leg_screw (Autodesk Fusion 360 design; units mm, degrees)
Autodesk Fusion 360 part; units mm, degrees
sketch "Sketch1" plane through (0, 0, 0) normal (0, 1, 0) x (1, 0, 0)
  circle A0 centre (0, 0) radius 10
  dimension "d1" = 20
  constraint coincident A0.centre origin
  measures "d1" diameter of A0
extrude "Extrude1" add sketch "Sketch1" along normal blind 3
sketch "Sketch2" plane through (0, 0, 0) normal (0, -1, 0) x (1, 0, 0)
  circle A0 centre (0, 0) radius 10
  circle A1 centre (0, 0) radius 4
  dimension "d4" = 8
  constraint coincident A0.centre A1.centre
  measures "d4" diameter of A1
extrude "Extrude2" add sketch "Sketch2" along normal blind 20 contours A1
thread "Thread1" "ISO Metric profile 8.0 M8x1.25 6g" major diameter 7.866 minor diameter 6.4455 pitch 1.25 angle 60 modelled right hand crest width 0.1833 on face at (3.995, -13.3333, -0.1994) crest through (3.933, 0.3125, 0)
sketch "Sketch4" plane through (0, 0, 0) normal (0, 0, 1) x (1, 0, 0)
  line L0 (-10, 3) -> (10, 3)
  line L1 (5, 3) -> (-5, 3)
  line L2 (-5, 3) -> (-5, 1.6)
  line L3 (-5, 1.6) -> (5, 1.6)
  line L4 (5, 1.6) -> (5, 3)
  dimension "d9" = 5
  dimension "d10" = 5
  dimension "d11" = 1.4
  constraint horizontal L0
  constraint horizontal L1
  constraint vertical L2
  constraint horizontal L3
  constraint vertical L4
  constraint coincident L0 L1.start
  measures "d9" horizontal distance of origin L1.end
  measures "d10" horizontal distance of origin L1.start
  measures "d11" distance of L1.end L2.end
extrude "Extrude3" cut sketch "Sketch4" along normal mid plane 1.5
pattern_circular "C-Pattern1" count 3 over 180 about axis through (0, 1.75, 0) along (0, 1, 0) of "Extrude3"
equation "d10 = d9"
equation "d12 = ( 1.5 / 2 ) * 1 mm"
